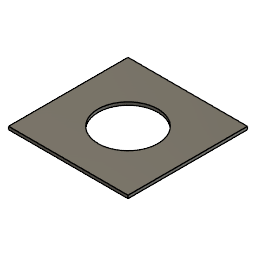
Day 13 Desgin Intent Washers (Autodesk Fusion 360 design; units mm, degrees)
part number: 2026-07-18-12-24-49-463
part number: 2026-07-18-12-27-19-294
part number: 2026-07-18-12-34-59-781
Autodesk Fusion 360 part; units mm, degrees
sketch "Sketch1" plane through (0, 0, 0) normal (0, 1, 0) x (1, 0, 0) in component "Design Intent 1"
  line L0 (100, 100) -> (-100, 100)
  line L1 (-100, 100) -> (-100, -100)
  line L2 (-100, -100) -> (100, -100)
  line L3 (100, -100) -> (100, 100)
  line L4 (100, 100) -> (-100, -100) construction
  line L5 (-100, 100) -> (100, -100) construction
  circle A0 centre (0, 0) radius 50
  dimension "d1" = 200
  dimension "d2" = 100
  constraint horizontal L0
  constraint perpendicular L0 L1
  constraint parallel L0 L2
  constraint parallel L1 L3
  constraint coincident L4 A0.centre
  constraint coincident L5 A0.centre
  constraint coincident A0.centre origin
  constraint equal L0 L1
  measures "d1" distance of L0.start L2.end
  measures "d2" diameter of A0
extrude "Extrude1" add sketch "Sketch1" along normal blind 5 makes body 1 in component "Design Intent 1"
sketch "Sketch1 (2)" plane through (0, 0, 0) normal (0, 1, 0) x (1, 0, 0) in component "Design Intent 2"
  line L0 (75, 75) -> (-75, 75)
  line L1 (-75, 75) -> (-75, -75)
  line L2 (-75, -75) -> (75, -75)
  line L3 (75, -75) -> (75, 75)
  line L4 (75, 75) -> (-75, -75) construction
  line L5 (-75, 75) -> (75, -75) construction
  circle A0 centre (0, -35) radius 25
  dimension "d1_1" = 150
  dimension "d2_1" = 50
  dimension "d5" = 40
  constraint horizontal L0
  constraint perpendicular L0 L1
  constraint parallel L0 L2
  constraint parallel L1 L3
  constraint coincident L4 origin
  constraint coincident L5 origin
  constraint equal L0 L1
  constraint vertical origin A0.centre
  measures "d1_1" distance of L0.start L2.end
  measures "d2_1" diameter of A0
  measures "d5" distance of L2 A0.centre
extrude "Extrude2" add sketch "Sketch1 (2)" along normal blind 5 separate body makes body 2 in component "Design Intent 1"
extrude "Extrude2'" add sketch "Sketch1 (2)" along normal blind 5 separate body makes body 3 in component "Design Intent 2"
extrude "Extrude1'" add sketch "Sketch1 (2)" along normal blind 5 separate body makes body 4 in component "Design Intent 2"
component "Design Intent 1" placed x (1, 0, 0) y (0, 1, 0) z (0, 0, 1) at (0, 0, 0)
component "Design Intent 2" placed x (1, 0, 0) y (0, 1, 0) z (0, 0, 1) at (0, 0, 0)
hidden bodies 2
equation "d2 = d1 / 2"
